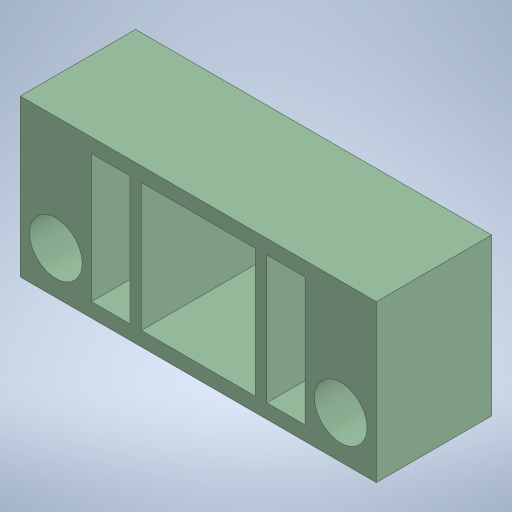
# Autodesk Inventor part: griper_base_TPU-2
Saved by Autodesk Inventor 2024 (Build 280153000, 153)
## iProperties
Created: 2025-06-06
Part Number: griper_base_TPU-2
Material: ゴム、シリコーン
Document SubType Name: Modeling
Designer: 1412z
Density: 1.25 g/cm^3
Appearance: ゴム - 緑
Author: 1412z
Autodesk Inventor part; units mm, degrees
ref_plane "YZ Plane" through (0, 0, 0) normal (1, 0, 0) x (0, 1, 0)
ref_plane "XZ Plane" through (0, 0, 0) normal (0, 1, 0) x (-1, 0, 0)
ref_plane "XY Plane" through (0, 0, 0) normal (0, 0, 1) x (1, 0, 0)
sketch "スケッチ1" plane through (0, 0, 0) normal (0, 0, 1) x (1, 0, 0)
  line L0 (12.5, -5.5) -> (-12.5, -5.5)
  line L1 (-12.5, -5.5) -> (-12.5, 5.5)
  line L2 (-12.5, 5.5) -> (12.5, 5.5)
  line L3 (12.5, 5.5) -> (12.5, -5.5)
  line L4 (12.5, -5.5) -> (-12.5, 5.5) construction
  line L5 (-12.5, -5.5) -> (12.5, 5.5) construction
  circle A0 centre (10, -2.5) radius 1.85
  circle A1 centre (-10, -2.5) radius 1.85
  line L6 (12.5, -4.5) -> (-12.5, -4.5)
  line L7 (12.5, 4.5) -> (-12.5, 4.5)
  line L8 (4, -4.5) -> (4, 4.5)
  line L9 (-4, -4.5) -> (-4, 4.5)
  line L10 (4.8, -4.5) -> (4.8, 4.5)
  line L11 (-4.8, -4.5) -> (-4.8, 4.5)
  line L12 (7.5, -4.5) -> (7.5, 4.5)
  line L13 (6.7, -4.5) -> (6.7, 4.5)
  line L14 (-7.5, -4.5) -> (-7.5, 4.5)
  line L15 (-6.7, -4.5) -> (-6.7, 4.5)
  point P0 (0, 0)
  dimension "d0" = 25
  dimension "d1" = 11
  dimension "d2" = 3.7
  dimension "d3" = 3.7
  constraints: 28 end point, 10 vertical, 4 point on line, 2 centre point, 2 midpoint, 2 parallel, 1 horizontal, 1 perpendicular, 22 other
  measures "d0" distance of L1.end L2.end
  measures "d1" distance of L0.end L1.end
  measures "d2" diameter of A0
  measures "d3" diameter of A1
extrude "押し出し1" add sketch "スケッチ1" along normal blind 8.1 contours L0 L1 L6 L3 | L6 L12 L7 L3 | L1 L7 L14 L6 | L7 L1 L2 L3 | L6 L8 L7 L10 | L11 L7 L9 L6
